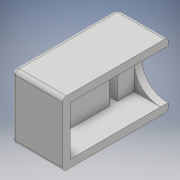
# Autodesk Inventor part: Support servomoteur
Saved by Autodesk Inventor 2017 (Build 210142000, 142)
## iProperties
Part Number: Support servomoteur
Material: Générique
Document SubType Name: Modeling
Designer: Geoff
Density: 1 g/cm^3
Appearance: Par défaut
Author: Geoff
Autodesk Inventor part; units mm, degrees
ref_plane "YZ Plane" through (0, 0, 0) normal (1, 0, 0) x (0, 1, 0)
ref_plane "XZ Plane" through (0, 0, 0) normal (0, 1, 0) x (-1, 0, 0)
ref_plane "XY Plane" through (0, 0, 0) normal (0, 0, 1) x (1, 0, 0)
sketch "Esquisse1" plane through (0, 0, 0) normal (1, 0, 0) x (0, 1, 0)
  line L0 (0, 0) -> (28, 0)
  line L1 (28, 0) -> (28, -17)
  line L2 (28, -17) -> (0, -17)
  line L3 (0, -17) -> (0, 0)
  line L4 (0, 0) -> (0, -2)
  line L5 (0, -2) -> (2, -2)
  line L6 (28, -17) -> (28, -15)
  line L7 (28, -15) -> (26, -15)
  line L8 (26, -15) -> (2, -15)
  line L9 (2, -15) -> (2, -2)
  line L10 (2, -2) -> (26, -2)
  line L11 (26, -2) -> (26, -15)
  dimension "d1" = 28
  dimension "d2" = 17
  dimension "d3" = 2
  dimension "d4" = 2
  dimension "d5" = 2
  dimension "d6" = 2
  constraints: 24 end point, 4 parallel, 4 perpendicular, 2 horizontal, 2 point on line
  measures "d1" distance of L1.end L2.end
  measures "d2" distance of L0.end L1.end
  measures "d3" distance of L0.start L4.end
  measures "d4" distance of L4.end L5.end
  measures "d5" distance of L1.end L6.end
  measures "d6" distance of L6.end L7.end
extrude "Extrusion1" add sketch "Esquisse1" along normal blind 13.5 contours L0 L1 L7 L11 L10 L5 L3 | L5 L9 L8 L7 L1 L2 L3
sketch "Esquisse2" plane through (0, 0, 0) normal (-1, 0, 0) x (0, 0, 1)
  line L0 (-2, 2) -> (-2, 26) projected
  line L1 (-2, 26) -> (-15, 26)
  line L2 (-15, 26) -> (-15, 2)
  line L3 (-15, 2) -> (-2, 2)
  line L4 (-2, 2) -> (-2, 26)
  point P0 (0, 0)
  constraints: 8 end point, 2 parallel, 1 horizontal, 1 perpendicular
extrude "Extrusion2" add sketch "Esquisse2" against normal blind 2
sketch "Esquisse3" plane through (2, 0, 0) normal (1, 0, 0) x (0, 0, -1)
  line L0 (15, 2) -> (2, 2) projected
  line L1 (2, 2) -> (2, 19.4)
  line L2 (2, 2) -> (2, 26) projected
  line L3 (2, 19.4) -> (2, 21.5)
  line L4 (2, 21.5) -> (2, 26)
  line L5 (2, 21.5) -> (2, 26)
  line L6 (15, 2) -> (2, 2)
  line L7 (2, 2) -> (2, 19.4)
  line L8 (2, 19.4) -> (15, 19.4)
  line L9 (15, 19.4) -> (15, 2)
  line L10 (2, 26) -> (15, 26) projected
  line L11 (15, 26) -> (2, 26)
  line L12 (2, 26) -> (2, 21.5)
  line L13 (2, 21.5) -> (15, 21.5)
  line L14 (15, 21.5) -> (15, 26)
  point P0 (0, 0)
  dimension "d11" = 17.4
  dimension "d12" = 2.1
  constraints: 24 end point, 4 parallel, 2 collinear, 2 horizontal, 2 perpendicular, 2 point on line
  measures "d11" distance of L0.end L1.end
  measures "d12" distance of L1.end L3.end
extrude "Extrusion3" add sketch "Esquisse3" along normal blind 4.5
sketch "Esquisse4" plane through (6.5, 0, 0) normal (1, 0, 0) x (0, 0, -1)
  line L0 (15, 2) -> (2, 2) projected
  line L1 (15, 2) -> (2, 2)
  line L2 (2, 2) -> (2, 8)
  line L3 (2, 8) -> (15, 8)
  line L4 (15, 8) -> (15, 2)
  point P0 (0, 0)
  dimension "d15" = 6
  constraints: 8 end point, 2 parallel, 1 horizontal, 1 perpendicular
  measures "d15" distance of L1.end L2.end
extrude "Extrusion4" cut sketch "Esquisse4" against normal blind 2
sketch "Esquisse5" plane through (13.5, 26, -15) normal (0, -1, 0) x (1, 0, 0)
  line L0 (-9, 13) -> (0, 13) projected
  line L1 (-9, 0) -> (0, 0) projected
  arc A0 (0, 13) -> (0, 0) centre (-0.4821, 6.5) ccw
  line L2 (0, 0) -> (0, 13) projected
  line L3 (0, 13) -> (0, 0)
  point P0 (-13.5, 15)
  constraints: 2 end point, 2 point on circle, 1 centre point, 1 perpendicular
extrude "Extrusion5" cut sketch "Esquisse5" against normal up to next
fillet "Congé1" radius 1 1 edges at (0, 14, 0)
fillet "Congé2" radius 1 1 edges at (0, 14, -17)
fillet "Congé3" radius 1 5 edges at (0.2929, 28, -0.2929) (7.25, 28, 0) (0.2929, 28, -16.7071) (7.25, 28, -17) (0, 28, -8.5)
fillet "Congé4" radius 1 5 edges at (0.2929, 0, -16.7071) (7.25, 0, -17) (0.2929, 0, -0.2929) (7.25, 0, 0) (0, 0, -8.5)
